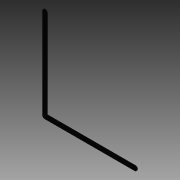
# Autodesk Inventor part: suelo_pruebas
Saved by Autodesk Inventor 2015 (Build 190159000, 159)
## iProperties
Created: 2015-06-07
Part Number: suelo_pruebas
Material: Genérico
Document SubType Name: Modeling
Designer: david_000
Density: 1 g/cm^3
Appearance: Textura fina - Negro
Author: david_000
Autodesk Inventor part; units mm, degrees
ref_plane "YZ Plane" through (0, 0, 0) normal (1, 0, 0) x (0, 1, 0)
ref_plane "XZ Plane" through (0, 0, 0) normal (0, 1, 0) x (-1, 0, 0)
ref_plane "XY Plane" through (0, 0, 0) normal (0, 0, 1) x (1, 0, 0)
sketch "Boceto1" plane through (0, 0, 0) normal (0, 1, 0) x (-1, 0, 0)
  line L0 (0, 0) -> (1000, 0)
  line L1 (1000, 25) -> (1000, 1000)
  line L2 (975, 1000) -> (975, 25)
  line L3 (975, 25) -> (0, 25)
  line L4 (1025, 1000) -> (1025, 0)
  line L5 (1000, -25) -> (0, -25)
  line L6 (1025, 1000) -> (975, 1000)
  line L7 (0, -25) -> (0, 25)
  circle A0 centre (0, 0) radius 25
  circle A1 centre (1000, 1000) radius 25
  arc A2 (1000, -25) -> (1025, 0) centre (1000, 0) ccw
  constraints: 16 end point, 4 perpendicular, 3 coincident, 2 horizontal, 2 point on circle, 1 centre point, 1 horizontal alignment, 1 tangent, 1 vertical alignment, 4 other
extrude "Extrusión1" add sketch "Boceto1" along normal blind 10
